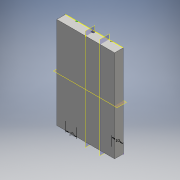
# Autodesk Inventor part: Circuit Board
Saved by Autodesk Inventor 2016 (Build 200138000, 138)
## iProperties
Created: 2016-05-06
Part Number: Circuit Board
Material: Generic
Document SubType Name: Modeling
Designer: Kenneth Daniel
Density: 1 g/cm^3
Appearance: Default
Author: Kenneth Daniel
Autodesk Inventor part; units mm, degrees
ref_plane "YZ Plane" through (0, 0, 0) normal (1, 0, 0) x (0, 1, 0)
ref_plane "XZ Plane" through (0, 0, 0) normal (0, 1, 0) x (-1, 0, 0)
ref_plane "XY Plane" through (0, 0, 0) normal (0, 0, 1) x (1, 0, 0)
sketch "Sketch1" plane through (0, 0, 0) normal (0, 1, 0) x (-1, 0, 0)
  line L0 (-25.2, 40) -> (-25.2, -40)
  line L1 (-25.2, -40) -> (25.2, -40)
  line L2 (25.2, -40) -> (25.2, 40)
  line L3 (25.2, 40) -> (-25.2, 40)
  line L4 (-25.2, 40) -> (25.2, -40) construction
  line L5 (-25.2, -40) -> (25.2, 40) construction
  point P0 (0, 0)
  dimension "d0" = 80
  dimension "d1" = 50.4
  constraints: 12 end point, 2 midpoint, 2 parallel, 1 perpendicular, 1 vertical
  measures "d0" distance of L0.start L0.end
  measures "d1" distance of L1.end L0.end
extrude "Extrusion1" add sketch "Sketch1" along normal blind 7.5
sketch "Sketch2" plane through (0, 7.5, 0) normal (0, 1, 0) x (1, 0, 0)
  line L0 (25.2, 40) -> (-25.2, 40) projected
  line L1 (-25.2, 40) -> (-15.2, 40)
  line L2 (-15.2, 40) -> (-15.2, -40)
  line L3 (-25.2, -40) -> (25.2, -40) projected
  line L4 (0, 40) -> (0, -40)
  line L5 (25.2, 40) -> (15.2, 40)
  line L6 (15.2, 40) -> (15.2, -40)
  line L7 (-14.2233, -40) -> (-14.2233, 40)
  line L8 (-14.2233, 40) -> (-16.1767, 40)
  line L9 (-16.1767, 40) -> (-16.1767, -40)
  line L10 (-16.1767, -40) -> (-14.2233, -40)
  line L11 (-14.2233, -40) -> (-16.1767, 40) construction
  line L12 (-14.2233, 40) -> (-16.1767, -40) construction
  point P0 (0, 0)
  point P1 (-15.2, 0)
  dimension "d4" = 10
  dimension "d5" = 10
  constraints: 22 end point, 5 midpoint, 4 point on line, 3 parallel, 3 perpendicular
  measures "d4" distance of L0.end L1.end
  measures "d5" distance of L0.start L5.end
sketch "Sketch3" plane through (-25.2, 0, 40) normal (0, 0, 1) x (1, 0, 0)
  point P0 (25.2, 0)
sketch "Sketch4" plane through (-25.2, 0, 40) normal (0, 0, 1) x (1, 0, 0)
  line L0 (0, 7.5) -> (50.4, 7.5) projected
  line L1 (9.0233, 7.5) -> (10.9782, 7.5)
  line L2 (9.0233, 7.5) -> (10.0298, 6.523)
  line L3 (10.0298, 6.523) -> (10.9782, 7.5)
  point P0 (25.2, 0)
  constraints: 6 end point, 2 point on line, 1 perpendicular
extrude "Extrusion2" cut sketch "Sketch4" against normal up to surface (80 mm away)
ref_plane "Work Plane1" through (0, 0, -40) normal (-1, 0, 0) x (0, 0, 1)
mirror "Mirror1" about plane through (0, 0, -40) normal (-1, 0, 0) of "Extrusion2"
ref_plane "Work Plane2" through (12.6, 0, -40) normal (-1, 0, 0) x (0, 0, 1)
sketch "Sketch5" plane through (25.2, 0, -40) normal (0, 0, -1) x (-1, 0, 0)
  line L0 (39.4218, 7.5) -> (10.9782, 7.5) projected
  line L1 (25.2, 7.5) -> (24.2, 7.5)
  line L2 (24.2, 7.5) -> (24.2, 5.5)
  line L3 (24.2, 5.5) -> (26.2, 5.5)
  line L4 (26.2, 5.5) -> (26.2, 7.5)
  line L5 (24.2, 7.5) -> (26.2, 7.5)
  point P0 (25.2, 0)
  dimension "d8" = 1
  dimension "d9" = 2
  dimension "d10" = 2
  constraints: 10 end point, 3 perpendicular, 2 point on line, 1 collinear, 1 midpoint
  measures "d8" distance of L1.start L1.end
  measures "d9" distance of L1.end L2.end
  measures "d10" distance of L2.end L3.end
extrude "Extrusion3" cut sketch "Sketch5" against normal up to surface (80 mm away)
ref_plane "Work Plane3" through (-25.2, 0, 0) normal (0, 0, 1) x (1, 0, 0)
body "Solid1"
